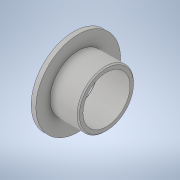
# Autodesk Inventor part: SKF_PPMF 101207
Saved by Autodesk Inventor 2022 (Build 260153000, 153)
## iProperties
Category: PARTsolutions
Company: SKF
Created: 2022-07-25
Part Number: SKF_PPMF 101207
Material: Generic
Catalog Web Link: www.cadenas.de
Description: BPR_A_F_B-Bushings
Vendor: SKF
Document SubType Name: Modeling
Designer: psAdmin
Manufacturer: SKF
Mass: 0.58 g
Surface Area: 8.44392 cm^2
Volume: 0.381114 cm^3
Density: 1 g/cm^3
Appearance: PSOLRGB-175-175-175
PSOL_IDENT_0: {$CADENAS_DATA/23d-libs/skf/bearings_units_and_housings/plain_bearings/bushings_washers_and_strips/b
PSOL_IDENT_1: pr_a_f_b.prj},177 {VTYP=3D},{NB=SKF_PPMF 101207},{LINA=SKF_PPMF 101207},{NN=BPR_A_F_B},{DATE=08.07.2
PSOL_IDENT_2: 022 10:25:42},{GEOMDATE=04.07.2022 06:52:09},{VERSION=},{LINEID=242390},{WBVAR=},{WBNUMERIC=}  {NB=S
PSOL_IDENT_3: KF_PPMF 101207},{LINA=SKF_PPMF 101207},{KT=DUMMY},{DESIGNATION=PPMF 101207},{DESIGN2=bushing_ppmf},{
PSOL_IDENT_4: DD=10.000},{D=12.000},{B=7.000},{D1=18},{AA=},{HH=},{ALPHA=},{MASS=0.00058},{CC1=0.000},{CC2=0.000},
PSOL_IDENT_5: {CHF1=0.000},{CHF2=0.000},{CHF3=0.500},{B1=1},{M=},{LOAD1=},{LOAD2=},{LOAD3=},{LOAD4=},{BTAL=0.2},{R
PSOL_IDENT_6: AL=0},{C1MIN=},{C1MAX=},{C2MIN=},{C2MAX=},{CHAMFER=},{RMAX=},{TSHAFT=h9},{THOUSING=H7},{HINT=},{SHAF
PSOL_IDENT_7: TMIN=},{SHAFTMAX=},{HOUSINGMIN=},{HOUSINGMAX=},{K=40},{K0=80},{KM=},{A=},{VMIN=},{VMAX=1},{UMIN=0.06
PSOL_IDENT_8: },{UMAX=0.15},{AAA=},{TEMPMIN=-30},{TEMPMAX=110},{BUSHING=PPMF 101207},{POPULAR=},{AAALG=0.000},{D1A
PSOL_IDENT_9: LG=18.000},{MALG=0.000},{HHALG=0.000},{B1ALG=1.000},{ALPHAALG=0.000},{DESIGN=Flanged}
NB: SKF_PPMF 101207
NN: BPR_A_F_B
NT: Bushings
NBSYN: SKF_$DESIGNATION.
LINA: SKF_PPMF 101207
CATALOG: SKF
DESIGNATION: PPMF 101207
DD: 10
D: 12
B: 7
D1: 18
DESIGN: Flanged
SUPPLIER: SKF
ARTICLENO: SKF_PPMF 101207
BOMINFO: SKF_PPMF 101207
CREATOR: CADENAS GmbH
Title: SKF_PPMF 101207
Author: Cadenas PARTsolutions
Comments: Bushings
Autodesk Inventor part; units mm, degrees
ref_plane "YZ Plane" through (0, 0, 0) normal (1, 0, 0) x (0, 1, 0)
ref_plane "XZ Plane" through (0, 0, 0) normal (0, 1, 0) x (-1, 0, 0)
ref_plane "XY Plane" through (0, 0, 0) normal (0, 0, 1) x (1, 0, 0)
sketch "Sketch_1" plane through (0, 0, 0) normal (0, 0, 1) x (1, 0, 0)
  line L0 (7, 0) -> (0, 0)
  line L1 (0, 9) -> (0, 5.25)
  line L2 (0, 5.25) -> (0.25, 5)
  line L3 (0.25, 5) -> (7, 5)
  line L4 (7, 5) -> (7, 5.75)
  line L5 (7, 5.75) -> (6.75, 6)
  line L6 (6.75, 6) -> (1, 6)
  line L7 (1, 6) -> (1, 9)
  line L8 (1, 9) -> (0, 9)
  constraints: 18 end point
revolve "Revolution1" add sketch "Sketch_1" angle 360 about axis through (7, 0, 0) along (1, 0, 0)
body "Solid1"
